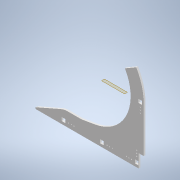
# Autodesk Inventor part: OuterWheelIndexer
Saved by Autodesk Inventor 2020 (Build 240168000, 168)
## iProperties
Created: 2020-01-19
Part Number: OuterWheelIndexer
Material: Generic
Document SubType Name: Modeling
Designer: srini
Density: 1 g/cm^3
Appearance: Default
Author: srini
Autodesk Inventor part; units mm, degrees
ref_plane "YZ Plane" through (0, 0, 0) normal (1, 0, 0) x (0, 1, 0)
ref_plane "XZ Plane" through (0, 0, 0) normal (0, 1, 0) x (-1, 0, 0)
ref_plane "XY Plane" through (0, 0, 0) normal (0, 0, 1) x (1, 0, 0)
sketch "Sketch1" plane through (0, 0, 0) normal (0, 0, 1) x (1, 0, 0)
  arc A0 (214.793, 155.575) -> (-1.2995, -306.5385) centre (-54.6708, 0) ccw
  line L0 (-1.2995, -306.5385) -> (-100.7285, -323.85)
  line L1 (-189.1562, -406.4) -> (313.6292, -406.4)
  line L2 (351.7292, -406.4) -> (351.7292, 0)
  arc A1 (-1.2995, -306.5385) -> (214.793, 155.575) centre (-54.6708, 0) ccw
  line L3 (-54.6708, 0) -> (401.7178, 0) construction
  arc A2 (351.7292, 0) -> (297.2819, 203.2) centre (-54.6708, 0) ccw
  line L4 (297.2819, 203.2) -> (214.793, 155.575)
  line L5 (34.2292, -406.4) -> (59.6292, -406.4)
  line L6 (59.6292, -406.4) -> (59.6292, -381)
  line L7 (59.6292, -381) -> (34.2292, -381)
  line L8 (34.2292, -381) -> (34.2292, -406.4)
  line L9 (288.2292, -406.4) -> (351.7292, -406.4)
  line L10 (313.6292, -406.4) -> (313.6292, -381)
  line L11 (313.6292, -381) -> (288.2292, -381)
  line L12 (288.2292, -381) -> (288.2292, -406.4)
  circle A3 centre (-54.6708, 0) radius 200.5558 construction
  line L13 (313.6292, 12.7) -> (339.0292, 12.7)
  line L14 (339.0292, 12.7) -> (339.0292, -12.7)
  line L15 (339.0292, -12.7) -> (313.6292, -12.7)
  line L16 (313.6292, -12.7) -> (313.6292, 12.7)
  line L17 (313.6292, 12.7) -> (339.0292, -12.7) construction
  line L18 (339.0292, 12.7) -> (313.6292, -12.7) construction
  line L19 (-189.1562, -406.4) -> (-358.8569, -425.45)
  line L20 (-358.8569, -425.45) -> (351.7292, -425.45)
  line L21 (351.7292, -425.45) -> (351.7292, -406.4)
  line L22 (313.6292, -406.4) -> (351.7292, -406.4)
  line L23 (-358.8569, -425.45) -> (-100.7285, -323.85)
  line L24 (-100.7285, -323.85) -> (-227.7285, -323.85)
  line L25 (-227.7285, -323.85) -> (-460.4569, -425.45)
  line L26 (-460.4569, -425.45) -> (-358.8569, -425.45)
  line L27 (-245.1708, -381) -> (-219.7708, -381)
  line L28 (-219.7708, -381) -> (-219.7708, -406.4)
  line L29 (-219.7708, -406.4) -> (-245.1708, -406.4)
  line L30 (-245.1708, -406.4) -> (-245.1708, -381)
  line L31 (-100.7285, -323.85) -> (-189.1562, -406.4)
  point P0 (290.2482, -355.6)
  point P1 (326.3292, 0)
  point P2 (326.3292, 0)
  point P3 (302.9482, -330.2)
  point P4 (298.4754, -355.6)
  point P5 (302.9482, -12.7)
  point P6 (302.7291, 12.7)
  point P7 (-245.1708, -386.8886)
  point P8 (-227.8836, -381)
  dimension "d0" = 622.3
  dimension "d1" = 406.4
  dimension "d2" = 30
  dimension "d4" = 406.4
  dimension "d7" = 25.4
  dimension "d8" = 25.4
  dimension "d9" = 38.1
  dimension "d10" = 292.1
  dimension "d21" = 25.4
  dimension "d22" = 25.4
  dimension "d23" = 25.4
  dimension "d27" = 19.05
  dimension "d32" = 101.6
  dimension "d33" = 101.6
  dimension "d40" = 254
  dimension "d41" = 127
  constraints: 64 end point, 10 parallel, 8 horizontal, 7 point on line, 6 point on circle, 4 perpendicular, 3 centre point, 3 equal length, 3 midpoint, 2 collinear, 2 concentric, 1 coincident, 1 tangent, 1 vertical
  measures "d0" diameter of A0
  measures "d1" distance from line of L3.start L2
  measures "d2" angle of L3 L4
  measures "d4" distance between parallel lines of L1 L3
  measures "d7" distance of L6.end L7.end
  measures "d8" distance of L5.end L6.end
  measures "d9" distance between parallel lines of L10 L2
  measures "d10" distance between parallel lines of L6 L2
  measures "d21" distance of L13.start L13.end
  measures "d22" distance of L13.end L14.end
  measures "d23" distance from line of point (326.329, 0) L2
  measures "d27" distance between parallel lines of L20 L1
  measures "d32" distance of L25.end L19.end
  measures "d33" distance between parallel lines of L26 L24
  measures "d40" distance between parallel lines of L28 L8
  measures "d41" distance of L0.end L24.end
extrude "Extrusion1" add sketch "Sketch1" along normal blind 12.7 contours L4 A2 L2 L9 L10 L11 L12 L1 L6 L7 L8 L31 L0 A1 | L31 L19 L23 | L23 L26 L25 L24 | L19 L1 L9 L21 L20
ref_plane "Work Plane1" through (59.6292, 0, 0) normal (0, 1, 0) x (-1, 0, 0)
fillet "Fillet3" radius 127 2 edges at (-100.7285, -323.85, 6.35) (-227.7285, -323.85, 6.35)
fillet "Fillet3" radius 6.35 1 edges at (-460.4569, -425.45, 6.35)
sketch "Sketch3" plane through (59.6292, 0, 0) normal (0, 1, 0) x (-1, 0, 0)
  line L0 (314.8558, -44.45) -> (-86.2558, -44.45) construction
  line L1 (114.3, -44.45) -> (114.3, -0.9544) construction
  circle A0 centre (355.6, -69.85) radius 88.9
  point P0 (59.6292, 0)
  dimension "d17" = 25.4
  dimension "d18" = 177.8
  dimension "d19" = 241.3
  constraints: 2 end point, 1 centre point, 1 midpoint, 1 vertical
  measures "d17" distance from line of A0.centre L0
  measures "d18" diameter of A0
  measures "d19" distance from line of A0.centre L1
revolve "Revolution2" cut sketch "Sketch3" angle 360 about axis through (-54.6708, 0, -44.45) along (0, 0, 1)
sketch "Sketch4" plane through (0, 0, 12.7) normal (0, 0, 1) x (1, 0, 0)
  circle A0 centre (85.0292, -393.7) radius 3.3734 projected
  circle A1 centre (104.0792, -393.7) radius 3.3734 projected
  circle A2 centre (123.1292, -393.7) radius 3.3734 projected
  circle A3 centre (224.7292, -393.7) radius 3.3734 projected
  circle A4 centre (243.7792, -393.7) radius 3.3734 projected
  circle A5 centre (262.8292, -393.7) radius 3.3734 projected
  circle A6 centre (300.9292, -355.6) radius 3.3734 projected
  circle A7 centre (300.9292, -336.55) radius 3.3734 projected
  circle A8 centre (300.9292, -317.5) radius 3.3734 projected
  circle A9 centre (326.3292, -76.2) radius 3.3734 projected
  circle A10 centre (326.3292, -57.15) radius 3.3734 projected
  circle A11 centre (326.3292, -38.1) radius 3.3734 projected
  circle A12 centre (-156.2708, -393.7) radius 3.3734 projected
  circle A13 centre (-175.3208, -393.7) radius 3.3734 projected
  circle A14 centre (-194.3708, -393.7) radius 3.3734 projected
  point P0 (0, 0)
extrude "Extrusion2" cut sketch "Sketch4" against normal through all
sketch "Sketch5" plane through (0, 0, 12.7) normal (0, 0, 1) x (1, 0, 0)
  line L0 (351.7292, -425.45) -> (314.3912, -425.45)
  line L1 (314.3912, -425.45) -> (314.3912, -328.676)
  line L2 (314.3912, -328.676) -> (351.7292, -328.676)
  line L3 (351.7292, -328.676) -> (351.7292, -425.45)
  line L4 (314.3912, -331.851) -> (314.3912, -328.676) projected
  point P0 (0, 0)
  constraints: 8 end point, 2 parallel, 1 horizontal, 1 perpendicular
extrude "Extrusion3" cut sketch "Sketch5" against normal through all
body "Solid1"
